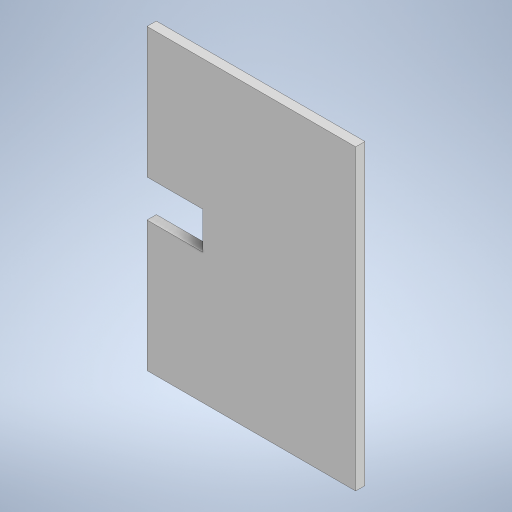
# Autodesk Inventor part: sadak_
Saved by Autodesk Inventor 2023 (Build 270158000, 158)
## iProperties
Created: 2023-02-13
Part Number: sadak_
Material: Generic
Document SubType Name: Modeling
Designer: Nikhil
Density: 1 g/cm^3
Appearance: Default
Author: Nikhil
Autodesk Inventor part; units mm, degrees
ref_plane "YZ Plane" through (0, 0, 0) normal (1, 0, 0) x (0, 1, 0)
ref_plane "XZ Plane" through (0, 0, 0) normal (0, 1, 0) x (-1, 0, 0)
ref_plane "XY Plane" through (0, 0, 0) normal (0, 0, 1) x (1, 0, 0)
sketch "Sketch1" plane through (0, 0, 0) normal (0, 0, 1) x (1, 0, 0)
  line L0 (0, 0) -> (112, 0)
  line L1 (112, 0) -> (112, 160)
  line L2 (112, 160) -> (0, 160)
  line L3 (0, 160) -> (0, 90)
  line L4 (0, 90) -> (30, 90)
  line L5 (30, 90) -> (30, 70)
  line L6 (30, 70) -> (0, 70)
  line L7 (0, 70) -> (0, 0)
  dimension "d0" = 112
  dimension "d1" = 160
  dimension "d2" = 70
  dimension "d3" = 30
  dimension "d4" = 20
  constraints: 16 end point, 7 perpendicular, 1 horizontal, 1 point on line
  measures "d0" distance of L0.start L0.end
  measures "d1" distance of L0.end L1.end
  measures "d2" distance of L2.end L3.end
  measures "d3" distance of L3.end L4.end
  measures "d4" distance of L4.end L5.end
extrude "Extrusion1" add sketch "Sketch1" along normal blind 5
body "Solid1"
